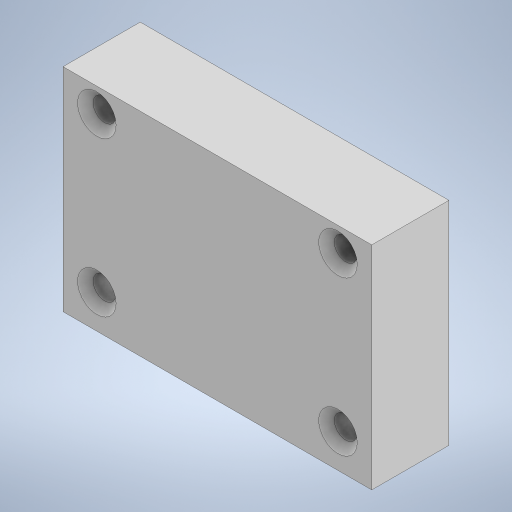
# Autodesk Inventor part: sensor_Mount
Saved by Autodesk Inventor 2023 (Build 270158000, 158)
## iProperties
Created: 2023-07-18
Part Number: sensor_Mount
Material: Generic
Document SubType Name: Modeling
Designer: checo
Density: 1 g/cm^3
Appearance: Default
Author: checo
Autodesk Inventor part; units mm, degrees
ref_plane "YZ Plane" through (0, 0, 0) normal (1, 0, 0) x (0, 1, 0)
ref_plane "XZ Plane" through (0, 0, 0) normal (0, 1, 0) x (-1, 0, 0)
ref_plane "XY Plane" through (0, 0, 0) normal (0, 0, 1) x (1, 0, 0)
sketch "Sketch1" plane through (0, 0, 0) normal (0, 0, 1) x (1, 0, 0)
  line L0 (0, 0) -> (0, 22)
  line L1 (0, 22) -> (32, 22)
  line L2 (32, 22) -> (32, 0)
  line L3 (32, 0) -> (0, 0)
  line L4 (16, 22) -> (16, 0) construction
  line L5 (32, 11) -> (0, 11) construction
  point P0 (3.5, 3.5)
  point P1 (28.5, 3.5)
  point P2 (3.5, 19.5)
  point P3 (28.5, 19.5)
  dimension "d0" = 32
  dimension "d1" = 22
  dimension "d2" = 3.5
  dimension "d3" = 3.5
  dimension "d4" = 2.5
  constraints: 12 end point, 4 midpoint, 3 perpendicular, 2 symmetric about line, 1 vertical, 1 vertical alignment
  measures "d0" distance of L2.end L0.start
  measures "d1" distance of L0.start L0.end
  measures "d2" distance from line of L0 point (3.5, 3.5)
  measures "d3" distance from line of L3 point (3.5, 3.5)
  measures "d4" distance from line of L1 point (3.5, 19.5)
extrude "Extrusion1" add sketch "Sketch1" against normal blind 8
hole "Hole1" at (3.5, 3.5, 0) at (28.5, 3.5, 0) at (3.5, 19.5, 0) at (28.5, 19.5, 0) direction (0, 0, -1) diameter 2.3813 depth 10 tip angle 118 countersink diameter 4 countersink angle 90
sketch "Sketch2" plane through (0, 0, -8) normal (0, 0, -1) x (-1, 0, 0)
  line L0 (-5.5, 1.75) -> (-26.5, 1.75)
  line L1 (-26.5, 1.75) -> (-26.5, 20.25)
  line L2 (-26.5, 20.25) -> (-5.5, 20.25)
  line L3 (-5.5, 20.25) -> (-5.5, 1.75)
  line L4 (-5.5, 1.75) -> (-26.5, 20.25) construction
  line L5 (-26.5, 1.75) -> (-5.5, 20.25) construction
  line L6 (-32, 22) -> (0, 22) projected
  line L7 (-16, 22) -> (-16, 0) construction
  line L8 (0, 0) -> (-32, 0) projected
  line L9 (-32, 0) -> (-32, 22) projected
  line L10 (-32, 11) -> (0, 11) construction
  line L11 (0, 22) -> (0, 0) projected
  point P0 (-16, 11)
  dimension "d14" = 21
  dimension "d15" = 18.5
  constraints: 16 end point, 7 midpoint, 2 parallel, 1 horizontal, 1 perpendicular
  measures "d14" distance of L1.end L2.end
  measures "d15" distance of L2.end L0.start
extrude "Extrusion2" cut sketch "Sketch2" against normal blind 3.5 contours L0 L1 L2 L3
sketch "Sketch3" plane through (0, 0, -8) normal (0, 0, -1) x (-1, 0, 0)
  point P0 (0, 0)
body "Solid1"
